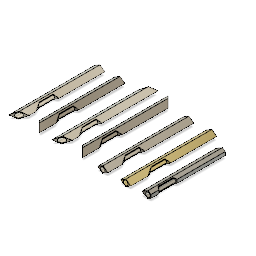
05-Pen Holders v1 (Autodesk Fusion 360 design; units mm, degrees)
Autodesk Fusion 360 part; units mm, degrees
note: some values were not read from the file. Set by a fixed rule: which sketch regions a step uses.
sketch "Sketch1" plane through (0, 0, 0) normal (0, 0, 1) x (1, 0, 0)
  line L0 (17.3205, 20) -> (34.641, 50)
  line L1 (34.641, 50) -> (17.3205, 80)
  line L2 (-34.641, 50) -> (-17.3205, 20)
  line L3 (-17.3205, 20) -> (17.3205, 20)
  line L4 (17.3205, 80) -> (0, 110)
  line L5 (-34.641, 50) -> (0, 110)
  circle A0 centre (0, 50) radius 22
  point P0 (0, 50)
  constraint parallel L1 L4
  constraint coincident P0 A0.centre
extrude "Extrude1" add sketch "Sketch1" against normal blind 450 makes body 1
sketch "Sketch2" plane through (0, 0, 0) normal (1, 0, 0) x (0, 0, -1)
  line L0 (0, 50) -> (0, 20)
  line L1 (0, 20) -> (450, 20)
  line L2 (450, 20) -> (450, 50)
  line L3 (450, 50) -> (0, 50)
  line L4 (25, 20) -> (37.5, 41.6506)
  line L5 (25, 20) -> (50, 20) construction
  line L6 (37.5, 41.6506) -> (187.5, 41.6506)
  line L7 (187.5, 41.6506) -> (200, 20)
  line L8 (200, 20) -> (25, 20)
  dimension "d3" = 25
  dimension "d4" = 60
  dimension "d5" = 150
  dimension "d6" = 120
  dimension "d7" = 25
  constraint horizontal L5
  constraint coincident L1 L4.start
  constraint parallel L3 L6
  measures "d3" distance of L4.start L4.end
  measures "d4" angle of L4 L5
  measures "d5" distance of L4.end L6.end
  measures "d6" angle of L6 L7
  measures "d7" distance of L6.end L7.end
move_body "Move1" bodies 1 to x (1, 0, 0) y (0, 1, 0) z (0, 0, 1) at (0, 0, 30)
extrude "Extrude2" cut sketch "Sketch2" along normal mid plane 120 contours L1 L4 L6 L7 L8 bodies 1
scale "Scale1" factor 0.3 about (0, 110, 30) bodies 1
move_body "Align1" bodies 1 to x (1, 0, 0) y (0, 1, 0) z (0, 0, 1) at (0, 0, -30)
move_body "Align2" bodies 1 to x (1, 0, 0) y (0, 1, 0) z (0, 0, 1) at (0, -83, 0)
scale "Scale2" factor 0.6 about (10.3923, 9, 0) bodies 1
extrude "Extrude3" add 1 faces at (7.203, 13.4978, -81) along direction (0, 0, -1) blind 39 on bodies 1 bodies 1
extrude "Extrude4" add 1 faces at (7.203, 13.4978, 0) along direction (0, 0, 1) blind 4 on bodies 1 bodies 1
extrude "Extrude5" add 1 faces at (7.203, 13.4978, -120) along direction (0, 0, -1) blind 6 on bodies 1 bodies 1
move_body "Move2" bodies 1 to x (1, 0, 0) y (0, 1, 0) z (0, 0, 1) at (0, 0, -4)
sketch "Sketch3" plane through (0, 0, 0) normal (0, 0, 1) x (1, 0, 0)
  line L0 (-15, 20) -> (-21.9282, 16)
  line L1 (-21.9282, 16) -> (-21.9282, 8)
  line L2 (-21.9282, 8) -> (-15, 4)
  line L3 (-15, 4) -> (-8.0718, 8)
  line L4 (-8.0718, 8) -> (-8.0718, 16)
  line L5 (-8.0718, 16) -> (-15, 20)
  circle A0 centre (-15, 12) radius 4
  line L6 (-40, 21) -> (-34, 12)
  line L7 (-46, 12) -> (-40, 21)
  line L8 (-46, 12) -> (-40, 3)
  line L9 (-40, 3) -> (-34, 12)
  circle A1 centre (-40, 12) radius 4
  point P0 (-15, 12)
  point P1 (-15, 12)
  constraint coincident P0 A0.centre
extrude "Extrude6" add sketch "Sketch3" against normal blind 130 separate body makes body 2 at (-11.0199, 11.6017, -43.3333) makes body 3 at (-36.0199, 11.6017, -43.3333)
delete_body "RemoveBody1" bodies 2
sketch "Sketch4" plane through (0, 0, 0) normal (1, 0, 0) x (0, 0, -1)
  line L0 (0, 12) -> (0, 3)
  line L1 (0, 3) -> (130, 3)
  line L2 (130, 3) -> (130, 12)
  line L3 (130, 12) -> (0, 12)
  line L4 (32.1244, 10) -> (55.9585, 10)
  line L5 (60, 3) -> (55.9585, 10)
  line L6 (60, 3) -> (68.0829, 3) construction
  line L7 (20, 3) -> (32.1244, 10)
  line L8 (20, 3) -> (34, 3) construction
  dimension "d22" = 7
  dimension "d30" = 120
  dimension "d31" = 30
  constraint perpendicular L0 L4
  constraint coincident L1 L5.start
  constraint coincident L1 L7.start
  constraint horizontal L6
  constraint horizontal L8
  measures "d22" distance of L1 L4
  measures "d30" angle of L5 L6
  measures "d31" angle of L7 L8
extrude "Extrude7" cut sketch "Sketch4" against normal blind 128 contours L1 L4 L5 L7 bodies 3
extrude "Extrude8" add 1 faces at (-37.0226, 15.9069, 0) along direction (0, 0, 1) blind 5 on bodies 3 bodies 3
extrude "Extrude9" add 1 faces at (-37.0226, 15.9069, -130) along direction (0, 0, -1) blind 15 on bodies 3 bodies 3
extrude "Extrude10" cut 1 faces at (-37.0226, 15.9069, -145) along direction (0, 0, 1) blind 5 on bodies 3 bodies 3
extrude "Extrude11" add 1 faces at (-37.0226, 15.9069, 5) along direction (0, 0, 1) blind 5 on bodies 3 bodies 3
move_body "Align3" bodies 3 to x (0.5547, 0.83205, 0) y (-0.83205, 0.5547, 0) z (0, 0, 1) at (-15.3158, 31.6179, 0)
move_body "Align4" bodies 3 to x (1, 0, 0) y (0, 1, 0) z (0, 0, 1) at (0, 0, 0)
move_body "Align5" bodies 1 to x (1, 0, 0) y (0, 1, 0) z (0, 0, 1) at (0, -3.6, 0)
move_body "Align7" bodies 3 to x (1, 0, 0) y (0, 1, 0) z (0, 0, 1) at (0, 0, -10)
move_body "Move3" bodies 3 to x (0.866025, 0.5, 0) y (-0.5, 0.866025, 0) z (0, 0, 1) at (-0.9241, 23.4178, 0)
move_body "Move4" bodies 1 to x (0, 1, 0) y (-1, 0, 0) z (0, 0, 1) at (9.5569, 1.2431, 0)
copy_body "CopyPasteBodies1" bodies 3 makes body 4
move_body "Move5" bodies 4 to x (1, 0, 0) y (0, 1, 0) z (0, 0, 1) at (-40, 0, 0)
extrude "Extrude14" cut 1 faces at (-80.456, 6.7168, 0) along direction (0, 0, -1) blind 5 on bodies 4 bodies 4
move_body "Move6" bodies 4 to x (1, 0, 0) y (0, 1, 0) z (0, 0, 1) at (0, 0, 5)
extrude "Extrude15" add 1 faces at (-80.456, 6.7168, -145) along direction (0, 0, -1) blind 5 on bodies 4 bodies 4
copy_body "CopyPasteBodies2" bodies 3 makes body 5
move_body "Move7" bodies 5 to x (1, 0, 0) y (0, 1, 0) z (0, 0, 1) at (-75, 0, 0)
move_body "Move8" bodies 4 to x (1, 0, 0) y (0, 1, 0) z (0, 0, 1) at (10, 0, 0)
move_body "Move9" bodies 3 to x (1, 0, 0) y (0, 1, 0) z (0, 0, 1) at (10, 0, 0)
sketch "Sketch7" plane through (0, 0, 0) normal (0, 1, 0) x (1, 0, 0)
  line L0 (-110, 0) -> (-135, 25)
  line L1 (-135, 25) -> (-135, -10)
  line L2 (-135, -10) -> (-110, -10)
  line L3 (-110, -10) -> (-110, 0)
  constraint vertical L1
  constraint perpendicular L1 L2
  constraint perpendicular L2 L3
extrude "Extrude16" cut sketch "Sketch7" along normal mid plane 30 bodies 5
sketch "Sketch8" plane through (0, 0, 0) normal (0, 1, 0) x (1, 0, 0)
  line L0 (-110.5651, 70) -> (-110.5651, 150)
  line L1 (-128.5277, 18.5277) -> (-119.1603, 9.1603)
  line L2 (-119.1603, 9.1603) -> (-119.1603, 150)
  line L3 (-119.1603, 150) -> (-128.5277, 150)
  line L4 (-128.5277, 150) -> (-128.5277, 18.5277)
  line L5 (-110.5651, 150) -> (-119.1603, 150)
  line L6 (-110.5651, 150) -> (-128.5277, 150)
  line L7 (-128.5277, 150) -> (-128.5277, 167.9627)
  line L8 (-110.5651, 150) -> (-128.5277, 167.9627)
  dimension "d47" = 135
  constraint coincident L0.end L5.start
  constraint coincident L3.end L4.start
  constraint perpendicular L5 L7
  measures "d47" angle of L7 L8
extrude "Extrude17" add 1 faces at (-123.2536, 7.2197, -150) along direction (0, 0, -1) blind 25 separate body on bodies 5 makes body 6
extrude "Extrude18" cut sketch "Sketch8" along normal mid plane 38 contours L3 L5 L6 L7 L8 keep common part bodies 6
combine "Combine1" operation add target body 5 tool bodies 6
copy_body "CopyPasteBodies3" bodies 4 makes body 7
copy_body "CopyPasteBodies4" bodies 3 makes body 8
move_body "Move11" bodies 8 to x (1, 0, 0) y (0, 1, 0) z (0, 0, 1) at (-120, 0, 0)
sketch "Sketch9" plane through (0, 0, 0) normal (0, 1, 0) x (1, 0, 0)
  line L0 (-163.5277, 150) -> (-163.5277, 0)
  line L1 (-145.5651, 150) -> (-154.1603, 150)
  line L2 (-154.1603, 150) -> (-154.1603, 0)
  line L3 (-154.1603, 0) -> (-145.5651, 0)
  line L4 (-145.5651, 0) -> (-145.5651, 30)
  line L5 (-145.5651, 30) -> (-152.2502, 42.1244)
  line L6 (-152.2502, 42.1244) -> (-152.2502, 65.9585)
  line L7 (-152.2502, 65.9585) -> (-145.5651, 70)
  line L8 (-145.5651, 70) -> (-145.5651, 150)
  line L9 (-154.1603, 150) -> (-163.5277, 150)
  line L10 (-163.5277, 150) -> (-163.5277, 0)
  line L11 (-163.5277, 0) -> (-154.1603, 0)
  line L12 (-154.1603, 0) -> (-154.1603, 150)
  line L13 (-163.5277, 0) -> (-145.5651, 0)
  line L14 (-163.5277, 0) -> (-145.5651, 17.9627)
  line L15 (-145.5651, 17.9627) -> (-145.5651, 0)
  line L16 (-163.5277, 150) -> (-145.5651, 167.9627)
  line L17 (-145.5651, 167.9627) -> (-145.5651, 150)
  line L18 (-163.5277, 150) -> (-145.5651, 150)
  dimension "d52" = 135
  constraint coincident L0.end L10.end
  constraint coincident L3.end L4.start
  constraint coincident L4 L14.end
  constraint coincident L0.start L9.end
  constraint parallel L14 L16
  constraint coincident L1.start L8.end
  constraint perpendicular L1 L17
  constraint perpendicular L8 L18
  measures "d52" angle of L13 L14
extrude "Extrude19" cut sketch "Sketch9" along normal mid plane 30 contours L2 L11 L12 L13 L14 | L2 L3 L4 L12 L13 L14 L15 bodies 8
extrude "Extrude20" add 1 faces at (-150.456, 6.7168, -150) along direction (0, 0, -1) blind 26 separate body on bodies 8 makes body 9
extrude "Extrude21" cut sketch "Sketch9" along normal mid plane 36 contours L1 L9 L16 L17 L18 keep common part bodies 9
combine "Combine2" operation add target body 8 tool bodies 9
copy_body "CopyPasteBodies5" bodies 5 8 makes body 10 makes body 11
move_body "Move14" bodies 10 11 to x (1, 0, 0) y (0, 1, 0) z (0, 0, 1) at (-75, 0, 0)
sketch "Sketch11" plane through (0, 0, 0) normal (0, 1, 0) x (1, 0, 0)
  line L0 (-180, 180) -> (-250, 180)
  line L1 (-250, 180) -> (-250, 150)
  line L2 (-250, 150) -> (-180, 150)
  line L3 (-180, 150) -> (-180, 180)
  constraint horizontal L0
  constraint vertical L1
  constraint horizontal L2
  constraint vertical L3
extrude "Extrude28" cut sketch "Sketch11" along normal mid plane 20 bodies 10 11
